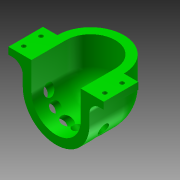
# Autodesk Inventor part: MotorShroud
Saved by Autodesk Inventor 2012 (Build 160160000, 160)
## iProperties
Created: 2013-08-15
Part Number: MotorShroud
Material: ABS Plastic
Document SubType Name: Modeling
Designer: joe_000
Density: 1.06 g/cm^3
Mass: 37.3697 g
Surface Area: 138.143 cm^2
Volume: 35.2544 cm^3
ShroudHoldShortSeperation: 0.500 in
ShroudHoldLongSeperation: 2.349 in
HoleDiameter: 0.118 in
Author: joe_000
Autodesk Inventor part; units mm, degrees
ref_plane "YZ Plane" through (0, 0, 0) normal (1, 0, 0) x (0, 1, 0)
ref_plane "XZ Plane" through (0, 0, 0) normal (0, 1, 0) x (-1, 0, 0)
sketch "Sketch1" plane through (0, 0, 0) normal (0, 0, 1) x (1, 0, 0)
  arc A0 (-18.127, 0) -> (18.127, 0) centre (0, 0) ccw
  arc A1 (-24.477, 0) -> (24.477, 0) centre (0, 0) ccw
  line L0 (-24.477, 0) -> (-24.477, 20.5)
  line L1 (24.477, 0) -> (24.477, 20.5)
  line L2 (-18.127, 0) -> (-18.127, 20.5)
  line L3 (18.127, 0) -> (18.127, 20.5)
  line L4 (24.477, 20.5) -> (18.127, 20.5)
  line L5 (-18.127, 20.5) -> (-24.477, 20.5)
  dimension "d1" = 36.254
  dimension "d2" = 6.35
  dimension "d3" = 20.5
  constraints: 12 end point, 6 perpendicular, 4 point on circle, 4 tangent, 2 centre point, 2 coincident, 2 parallel, 1 vertical
  measures "d1" diameter of A0
  measures "d2" radial gap between concentric circles of A0 A1
  measures "d3" distance of L1.start L1.end
extrude "Extrusion1" add sketch "Sketch1" along normal blind 25.4
sketch "Sketch2" plane through (18.127, 20.5, 0) normal (0, 1, 0) x (1, 0, 0)
  line L0 (6.35, 0) -> (6.35, -25.4) projected
  line L1 (6.35, 0) -> (0, 0) projected
  line L2 (6.35, 0) -> (16.921, 0)
  line L3 (16.921, 0) -> (16.921, -25.4)
  line L4 (16.921, -25.4) -> (6.35, -25.4)
  line L5 (6.35, -25.4) -> (6.35, 0)
  line L6 (0, -25.4) -> (6.35, -25.4) projected
  point P0 (-18.127, 0)
  point P1 (6.35, -12.7)
  dimension "d6" = 10.571
  constraints: 8 end point, 2 collinear, 2 parallel, 1 horizontal, 1 midpoint, 1 perpendicular, 1 point on line
  measures "d6" distance of L2.start L2.end
extrude "Extrusion2" add sketch "Sketch2" against normal blind 5.08
hole "Hole1" at (29.8379, 15.42, 19.3851) direction (0, 1, 0) diameter 3 end through all counterbore diameter 5.5 counterbore depth 0.0254
pattern_linear "Rectangular Pattern1" count 2 spacing 12.7 along (0, 0, -1) of "Hole1"
fillet "Fillet3" radius 7.62 1 edges at (24.477, 15.42, 12.7)
mirror "Mirror1" about plane through (0, 0, 0) normal (1, 0, 0) of "Extrusion2", "Hole1", "Rectangular Pattern1"
fillet "Fillet4" radius 7.62 1 edges at (-24.477, 15.42, 12.7)
sketch "Sketch6" plane through (0, 0, 0) normal (0, 0, -1) x (-1, 0, 0)
  arc A0 (-24.477, 0) -> (24.477, 0) centre (0, 0) ccw projected
  arc A1 (-18.127, 0) -> (18.127, 0) centre (0, 0) ccw projected
  line L0 (-18.127, 20.5) -> (-18.127, 0) projected
  line L1 (-24.477, 20.5) -> (-18.127, 20.5) projected
  line L2 (-24.477, 0) -> (-24.477, 20.5) projected
  line L3 (0, -18.127) -> (0, -24.477)
  constraints: 2 end point, 2 point on circle
revolve "Revolution1" add sketch "Sketch6" angle 180 about axis through (0, -18.127, 0) along (0, 1, 0)
sketch "Sketch7" plane through (0, 0, 25.4) normal (0, 0, 1) x (1, 0, 0)
  line L0 (-24.477, 0) -> (-24.477, 20.5) projected
  arc A0 (-24.477, 0) -> (24.477, 0) centre (0, 0) ccw projected
  line L1 (24.477, 20.5) -> (24.477, 0) projected
  line L2 (18.127, 20.5) -> (24.477, 20.5) projected
  line L3 (18.127, 0) -> (18.127, 20.5) projected
  arc A1 (-18.127, 0) -> (18.127, 0) centre (0, 0) ccw projected
  line L4 (-18.127, 20.5) -> (-18.127, 0) projected
  line L5 (-24.477, 20.5) -> (-18.127, 20.5) projected
  line L6 (0, 0) -> (-17.3079, -17.3079)
  line L7 (0, 0) -> (-18.127, 0)
  dimension "d38" = 45
  constraints: 4 end point, 1 parallel, 1 point on circle
  measures "d38" angle of L6 L7
ref_plane "Work Plane1" through (-17.3079, -17.3079, 25.4) normal (-0.7071068, -0.7071068, 0) x (0.7071068, -0.7071068, 0)
sketch "Sketch8" plane through (-17.3079, -17.3079, 25.4) normal (-0.7071068, -0.7071068, 0) x (0.7071068, -0.7071068, 0)
  line L0 (-17.3079, 0) -> (24.477, 0) projected
  circle A0 centre (-9.27, -12.238) radius 3.81
  circle A1 centre (9.27, -12.238) radius 3.81
  circle A2 centre (0, -12.238) radius 3.81
  point P0 (0, -25.4)
  point P1 (17.3079, 0)
  dimension "d49" = 7.62
  dimension "d50" = 9.27
  dimension "d51" = 9.27
  constraints: 3 centre point, 2 equal radius, 1 horizontal alignment
  measures "d49" diameter of A0
  measures "d50" horizontal distance of point (0, -25.4) A0.centre
  measures "d51" horizontal distance of A1.centre point (0, -25.4)
extrude "Extrusion3" cut sketch "Sketch8" against normal blind 19.05
mirror "Mirror2" about plane through (0, 0, 0) normal (1, 0, 0) of "Extrusion3"
sketch "Sketch9" plane through (35.048, 20.5, 25.4) normal (0, 1, 0) x (1, 0, 0)
  circle A0 centre (-5.2101, 6.0149) radius 1.5 projected
  circle A1 centre (-5.2101, 18.7149) radius 1.5 projected
  circle A2 centre (-64.8859, 18.7149) radius 1.5 projected
  circle A3 centre (-64.8859, 6.0149) radius 1.5 projected
  line L0 (-70.096, 0) -> (-53.175, 0) projected
  line L1 (-53.175, 25.4) -> (-53.175, 0) projected
  arc A4 (-16.921, 25.4) -> (-53.175, 25.4) centre (-35.048, 25.4) ccw projected
  line L2 (-16.921, 25.4) -> (-16.921, 0) projected
  line L3 (-16.921, 0) -> (0, 0) projected
  line L4 (0, 0) -> (0, 25.4) projected
  line L5 (0, 25.4) -> (-10.571, 25.4) projected
  arc A5 (-10.571, 25.4) -> (-59.525, 25.4) centre (-35.048, 25.4) ccw projected
  line L6 (-59.525, 25.4) -> (-70.096, 25.4) projected
  line L7 (-70.096, 0) -> (-70.096, 25.4) projected
  dimension "ShroudHoldLongSeperation" = 59.6758
  measures "ShroudHoldLongSeperation" distance of A0.centre A3.centre
equation "\"d3\" = MotorCenterOffset"
equation "\"MotorCenterOffset\" = 20.5"
body "Solid1"
